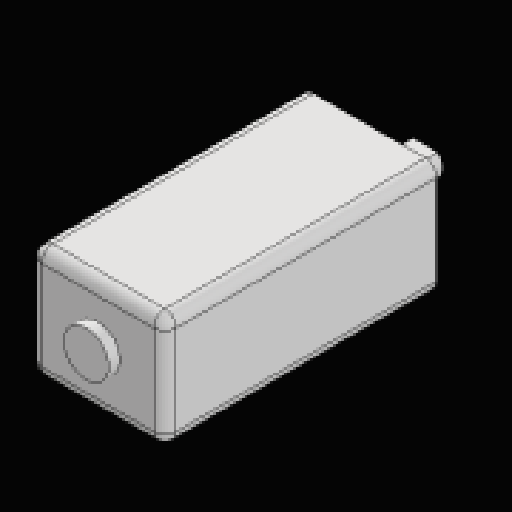
# Autodesk Inventor part: 1800rpm Brushed Motor
Saved by Autodesk Inventor 2023.2 (Build 272271030, 271C)
## iProperties
Created: 2023-11-10
Part Number: 1800rpm Brushed Motor
Material: Generic
Document SubType Name: Modeling
Designer: robpl
Density: 1 g/cm^3
Appearance: Default
Author: robpl
Autodesk Inventor part; units mm, degrees
ref_plane "YZ Plane" through (0, 0, 0) normal (1, 0, 0) x (0, 1, 0)
ref_plane "XZ Plane" through (0, 0, 0) normal (0, 1, 0) x (-1, 0, 0)
ref_plane "XY Plane" through (0, 0, 0) normal (0, 0, 1) x (1, 0, 0)
sketch "Sketch1" plane through (0, 0, 0) normal (0, 0, 1) x (1, 0, 0)
  line L0 (-6, 5) -> (6, 5)
  line L1 (6, 5) -> (6, -5)
  line L2 (6, -5) -> (-6, -5)
  line L3 (-6, -5) -> (-6, 5)
  line L4 (-6, 5) -> (6, -5) construction
  line L5 (6, 5) -> (-6, -5) construction
  point P0 (0, 0)
  dimension "d0" = 12
  dimension "d1" = 10
  constraints: 12 end point, 2 midpoint, 2 parallel, 1 horizontal, 1 perpendicular
  measures "d0" distance of L1.end L2.end
  measures "d1" distance of L0.end L1.end
extrude "Extrusion1" add sketch "Sketch1" along normal blind 24.25
sketch "Sketch2" plane through (0, 0, 24.25) normal (0, 0, 1) x (1, 0, 0)
  circle A0 centre (0, 0) radius 2
  dimension "d4" = 4
  constraints: 1 centre point, 1 coincident
  measures "d4" diameter of A0
extrude "Extrusion2" add sketch "Sketch2" along normal blind 1
sketch "Sketch3" plane through (0, 0, 0) normal (0, 0, -1) x (-1, 0, 0)
  circle A0 centre (0, 0) radius 2
  dimension "d7" = 4
  constraints: 1 centre point, 1 coincident
  measures "d7" diameter of A0
extrude "Extrusion3" add sketch "Sketch3" along normal blind 1
sketch "Sketch4" plane through (0, 0, -1) normal (0, 0, -1) x (-1, 0, 0)
  circle A0 centre (0, 0) radius 1.5
  line L0 (-1.5, 1) -> (1.5, 1)
  line L1 (1.5, 1) -> (1.5, -1.5)
  line L2 (1.5, -1.5) -> (-1.5, -1.5)
  line L3 (-1.5, -1.5) -> (-1.5, 1)
  point P0 (1.118, 1)
  point P1 (-1.118, 1)
  dimension "d10" = 3
  dimension "d11" = 2.5
  constraints: 8 end point, 3 tangent, 2 parallel, 1 centre point, 1 coincident, 1 horizontal, 1 perpendicular
  measures "d10" diameter of A0
  measures "d11" distance of L0.end L1.end
extrude "Extrusion4" add sketch "Sketch4" along normal blind 4 contours A0 L0 picked at (-0.0419, 0.0796)
fillet "Fillet1" radius 1 8 edges at (6, 5, 12.125) (-6, 5, 12.125) (6, -5, 12.125) (-6, -5, 12.125) (0, 5, 24.25) (6, 0, 24.25) (-6, 0, 24.25) (0, -5, 24.25)
sketch "Sketch5" plane through (0, 0, 0) normal (0, 0, -1) x (-1, 0, 0)
  arc A0 (5, -5) -> (6, -4) centre (5, -4) ccw projected
  line L0 (6, 4) -> (6, -4) projected
  arc A1 (6, 4) -> (5, 5) centre (5, 4) ccw projected
  line L1 (-5, 5) -> (5, 5) projected
  arc A2 (-5, 5) -> (-6, 4) centre (-5, 4) ccw projected
  line L2 (-6, -4) -> (-6, 4) projected
  arc A3 (-6, -4) -> (-5, -5) centre (-5, -4) ccw projected
  line L3 (5, -5) -> (-5, -5) projected
  circle A4 centre (0, 0) radius 2 projected
  point P0 (-4.5, 0)
  point P1 (4.5, 0)
  dimension "d15" = 4.5
  dimension "d16" = 4.5
  constraints: 2 horizontal alignment
  measures "d15" distance of point (-4.5, 0) point (0, 0)
  measures "d16" distance of point (4.5, 0) point (0, 0)
hole "Hole1" at (4.5, 0, 0) at (-4.5, 0, 0) direction (0, 0, 1) diameter 1.221 depth 1 thread size "M1.6x0.35" class "6H" standard "ISO Metric profile"
equation "\"d16\" = d15"
body "Solid1"
